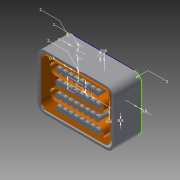
# Autodesk Inventor part: 4x8 arnyekolt vezetek
Saved by Autodesk Inventor 2015 (Build 190159000, 159)
## iProperties
Created: 2015-06-10
Part Number: 4x8 arnyekolt vezetek
Material: Generic
Document SubType Name: Modeling
Designer: laca
Density: 1 g/cm^3
Appearance: Default
Author: laca
Autodesk Inventor part; units mm, degrees
ref_plane "YZ Plane" through (0, 0, 0) normal (1, 0, 0) x (0, 1, 0)
ref_plane "XZ Plane" through (0, 0, 0) normal (0, 1, 0) x (-1, 0, 0)
ref_plane "XY Plane" through (0, 0, 0) normal (0, 0, 1) x (1, 0, 0)
sketch "Sketch1" plane through (0, 0, 0) normal (0, 0, 1) x (1, 0, 0)
  circle A0 centre (0, 0) radius 1
  line L0 (-11.2935, 0) -> (-8.6631, 0)
  line L1 (-8.6631, 0) -> (-11.2935, 0)
  line L2 (-11.2935, -2.7324) -> (-11.2935, -2.6412)
  line L3 (-11.2935, -2.6412) -> (-11.2935, 0)
  circle A1 centre (2, 0) radius 1
  circle A2 centre (4, 0) radius 1
  circle A3 centre (6, 0) radius 1
  circle A4 centre (8, 0) radius 1
  circle A5 centre (10, 0) radius 1
  circle A6 centre (12, 0) radius 1
  circle A7 centre (14, 0) radius 1
  circle A8 centre (0, 4) radius 1
  circle A9 centre (2, 4) radius 1
  circle A10 centre (4, 4) radius 1
  circle A11 centre (6, 4) radius 1
  circle A12 centre (8, 4) radius 1
  circle A13 centre (10, 4) radius 1
  circle A14 centre (12, 4) radius 1
  circle A15 centre (14, 4) radius 1
  circle A16 centre (0, 8) radius 1
  circle A17 centre (2, 8) radius 1
  circle A18 centre (4, 8) radius 1
  circle A19 centre (6, 8) radius 1
  circle A20 centre (8, 8) radius 1
  circle A21 centre (10, 8) radius 1
  circle A22 centre (12, 8) radius 1
  circle A23 centre (14, 8) radius 1
  circle A24 centre (0, 12) radius 1
  circle A25 centre (2, 12) radius 1
  circle A26 centre (4, 12) radius 1
  circle A27 centre (6, 12) radius 1
  circle A28 centre (8, 12) radius 1
  circle A29 centre (10, 12) radius 1
  circle A30 centre (12, 12) radius 1
  circle A31 centre (14, 12) radius 1
  line L4 (-0.8442, 14) -> (16.6577, 14)
  line L5 (16.6577, 8) -> (16.6577, 8)
  line L6 (14.6577, -2) -> (-4.0315, -2)
  line L7 (-2.8442, 12) -> (-2.8442, 12)
  line L8 (-0.8442, 10) -> (14.6577, 10)
  line L9 (-0.8442, 6) -> (14.6577, 6)
  line L10 (-0.8442, 2) -> (14.6577, 2)
  arc A32 (-0.8442, 14) -> (-2.8442, 12) centre (-0.8442, 12) ccw
  arc A33 (-2.8442, 12) -> (-0.8442, 10) centre (-0.8442, 12) ccw
  arc A34 (16.6577, 8) -> (14.6577, 10) centre (14.6577, 8) ccw
  arc A35 (14.6577, 6) -> (16.6577, 8) centre (14.6577, 8) ccw
  line L11 (-2.8442, 4) -> (-2.8442, 4)
  line L12 (16.6577, 0) -> (16.6577, 0)
  arc A36 (-0.8442, 6) -> (-2.8442, 4) centre (-0.8442, 4) ccw
  arc A37 (-2.8442, 4) -> (-0.8442, 2) centre (-0.8442, 4) ccw
  arc A38 (16.6577, 0) -> (14.6577, 2) centre (14.6577, 0) ccw
  arc A39 (14.6577, -2) -> (16.6577, 0) centre (14.6577, 0) ccw
  line L13 (-2.8442, -2) -> (-6.0315, -2)
  line L14 (-6.0315, 0) -> (-6.0315, 12.6)
  line L15 (-4.0315, 14.6) -> (16.8312, 14.6)
  line L16 (18.8312, 12.6) -> (18.8312, -0.6)
  line L17 (16.8312, -2.6) -> (-5.6626, -2.6)
  arc A40 (18.8312, 12.6) -> (16.8312, 14.6) centre (16.8312, 12.6) ccw
  arc A41 (-4.0315, 14.6) -> (-6.0315, 12.6) centre (-4.0315, 12.6) ccw
  arc A42 (-6.0315, 0) -> (-4.0315, -2) centre (-4.0315, 0) ccw
  arc A43 (16.8312, -2.6) -> (18.8312, -0.6) centre (16.8312, -0.6) ccw
  line L18 (-4.6315, 15.2) -> (17.4312, 15.2)
  line L19 (19.4312, 13.2) -> (19.4312, -1.2)
  line L20 (17.4312, -3.2) -> (-4.6315, -3.2)
  line L21 (-6.6315, -1.2) -> (-6.6315, 13.2)
  arc A44 (-4.6315, 15.2) -> (-6.6315, 13.2) centre (-4.6315, 13.2) ccw
  arc A45 (-6.6315, -1.2) -> (-4.6315, -3.2) centre (-4.6315, -1.2) ccw
  arc A46 (17.4312, -3.2) -> (19.4312, -1.2) centre (17.4312, -1.2) ccw
  arc A47 (19.4312, 13.2) -> (17.4312, 15.2) centre (17.4312, 13.2) ccw
  line L22 (-7.4315, 13.2) -> (-7.4315, -1.2)
  arc A48 (-7.4315, -1.2) -> (-4.6315, -4) centre (-4.6315, -1.2) ccw
  line L23 (-4.6315, -4) -> (17.4312, -4)
  arc A49 (17.4312, -4) -> (20.2312, -1.2) centre (17.4312, -1.2) ccw
  line L24 (20.2312, -1.2) -> (20.2312, 13.2)
  arc A50 (20.2312, 13.2) -> (17.4312, 16) centre (17.4312, 13.2) ccw
  line L25 (17.4312, 16) -> (-4.6315, 16)
  arc A51 (-4.6315, 16) -> (-7.4315, 13.2) centre (-4.6315, 13.2) ccw
  point P0 (16.6577, -2)
  point P1 (-2.8442, 6)
  point P2 (-2.8442, 2)
  point P3 (16.6577, 2)
  dimension "d0" = 2
  dimension "d3" = 2
  dimension "d6" = 4
  dimension "d9" = 2
  dimension "d10" = 4
  dimension "d11" = 4
  dimension "d12" = 4
  dimension "d13" = 2
  dimension "d14" = 2
  dimension "d15" = 2
  dimension "d16" = 2
  dimension "d17" = 2
  dimension "d18" = 0.6
  dimension "d19" = 0.6
  dimension "d20" = 0.6
  dimension "d21" = 0.6
  dimension "d22" = 0.6
  dimension "d23" = 0.6
  dimension "d24" = 0.8
  constraints: 52 centre point, 52 end point, 40 point on circle, 32 coincident, 32 tangent, 16 point on line, 12 equal radius, 10 parallel, 7 perpendicular, 5 horizontal, 3 vertical, 2 collinear, 100 other
  measures "d0" diameter of A0
  measures "d3" distance of point (0, 0) point (2, 0)
  measures "d6" distance of point (0, 0) point (0, 4)
  measures "d9" distance from line of L8 point (0, 12)
  measures "d10" distance between parallel lines of L9 L8
  measures "d11" distance between parallel lines of L10 L9
  measures "d12" distance between parallel lines of L6 L10
  measures "d13" distance from line of point (0, 12) L4
  measures "d14" radius of A32
  measures "d15" radius of A36
  measures "d16" radius of A40
  measures "d17" radius of A44
  measures "d18" distance between parallel lines of L21 L14
  measures "d19" distance between parallel lines of L19 L16
  measures "d20" distance between parallel lines of L20 L17
  measures "d21" distance between parallel lines of L15 L18
  measures "d22" distance between parallel lines of L4 L15
  measures "d23" distance between parallel lines of L17 L6
  measures "d24" distance between parallel lines of L22 L21
extrude "Extrusion1" add sketch "Sketch1" along normal blind 10
surface extrude "ExtrusionSrf1" sketch "Sketch1" along normal blind 10 shown yes curves L4 A32 L7 A33 L8 A34 L5 A35 L9 A36 L11 A37 L10 A38 L12 A39 L6 A42 L14 A41 L15 A40 L16 A43 L17
body "Solid1"
body "Srf1"
